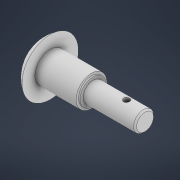
# Autodesk Inventor part: 4
Saved by Autodesk Inventor 2022 (Build 260153000, 153)
## iProperties
Created: 2022-09-05
Part Number: 4
Material: 일반
Document SubType Name: Modeling
Designer: USER
Density: 1 g/cm^3
Appearance: 기본값
Author: USER
Autodesk Inventor part; units mm, degrees
ref_plane "YZ Plane" through (0, 0, 0) normal (1, 0, 0) x (0, 1, 0)
ref_plane "XZ Plane" through (0, 0, 0) normal (0, 1, 0) x (-1, 0, 0)
ref_plane "XY Plane" through (0, 0, 0) normal (0, 0, 1) x (1, 0, 0)
sketch "스케치1" plane through (0, 0, 0) normal (0, 0, 1) x (1, 0, 0)
  line L0 (-84.1615, 0) -> (93.5573, 0)
  arc A0 (-68.0067, 18.4178) -> (-77.974, 0) centre (-55.974, 0) ccw
  line L1 (-68.0067, 0) -> (-41.0067, 0)
  line L2 (-41.0067, 0) -> (-41.0067, 10)
  line L3 (-41.0067, 10) -> (-68.0067, 10)
  line L4 (-68.0067, 10) -> (-68.0067, 0)
  line L5 (-39.974, 0) -> (-6.974, 0)
  line L6 (-6.974, 0) -> (-6.974, 6.5)
  line L7 (-6.974, 6.5) -> (-39.974, 6.5)
  line L8 (-39.974, 6.5) -> (-39.974, 0)
  line L9 (-68.0067, 10) -> (-68.0067, 18.4178)
  line L10 (-41.0067, 8.4887) -> (-39.974, 8.4887)
  line L11 (-39.974, 8.4887) -> (-39.974, 0)
  line L12 (-39.974, 0) -> (-41.0067, 0)
  line L13 (-41.0067, 0) -> (-41.0067, 8.4887)
  line L14 (-6.974, 0) -> (-5.974, 0)
  line L15 (-5.974, 0) -> (-5.974, 6.5)
  line L16 (-5.974, 6.5) -> (-6.974, 6.5)
  line L17 (-6.974, 6.5) -> (-6.974, 0)
  point P0 (0, 0)
  dimension "d0" = 22
  dimension "d1" = 71
  dimension "d2" = 27
  dimension "d3" = 33
  dimension "d4" = 20
  dimension "d5" = 13
  dimension "d6" = 13
  dimension "d7" = 1
  constraints: 36 end point, 8 parallel, 5 horizontal, 5 point on line, 4 perpendicular, 2 point on circle, 1 centre point, 1 vertical
  measures "d0" distance of A0.centre A0.end
  measures "d1" distance from line of L6 A0.end
  measures "d2" distance between parallel lines of L2 L4
  measures "d3" distance between parallel lines of L6 L8
  measures "d4" diameter of L3 L0
  measures "d5" diameter of L7 L0
  measures "d6" diameter of L16 L0
  measures "d7" distance between parallel lines of L15 L6
revolve "회전1" add sketch "스케치1" angle 360 about axis through (-84.1615, 0, 0) along (1, 0, 0)
chamfer "모따기1" distance 1 angle 45 1 edges at (-5.974, -6.5, 0)
sketch "스케치2" plane through (0, 0, 0) normal (0, 1, 0) x (-1, 0, 0)
  circle A0 centre (17.974, 0) radius 2
  line L0 (39.974, 8.4887) -> (39.974, -8.4887) projected
  point P0 (0, 0)
  dimension "d12" = 4
  dimension "d13" = 22
  constraints: 1 centre point
  measures "d12" diameter of A0
  measures "d13" distance from line of L0 A0.centre
extrude "돌출1" cut sketch "스케치2" along normal through all both and the other way through all
